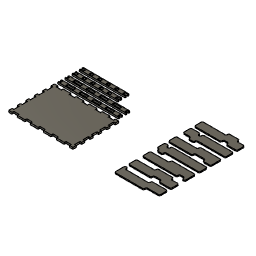
Púsl og Bakki (Autodesk Fusion 360 design; units mm, degrees)
Autodesk Fusion 360 part; units mm, degrees
(part 1 of 3)
sketch "Sketch1" plane through (0, 0, 0) normal (0, 0, 1) x (1, 0, 0)
  line L0 (0, 0) -> (121.4, 0)
  line L1 (121.4, 0) -> (121.4, 86.4)
  line L2 (121.4, 86.4) -> (0, 86.4)
  line L3 (0, 86.4) -> (0, 0)
  line L4 (6.4, 0) -> (16.4, 0)
  line L5 (16.4, 0) -> (16.4, 3.2)
  line L6 (16.4, 3.2) -> (6.4, 3.2)
  line L7 (6.4, 3.2) -> (6.4, 0)
  line L8 (31.05, 3.2) -> (31.05, 0)
  line L9 (41.05, 3.2) -> (31.05, 3.2)
  line L10 (31.05, 0) -> (41.05, 0)
  line L11 (41.05, 0) -> (41.05, 3.2)
  line L12 (55.7, 3.2) -> (55.7, 0)
  line L13 (65.7, 3.2) -> (55.7, 3.2)
  line L14 (55.7, 0) -> (65.7, 0)
  line L15 (65.7, 0) -> (65.7, 3.2)
  line L16 (80.35, 3.2) -> (80.35, 0)
  line L17 (90.35, 3.2) -> (80.35, 3.2)
  line L18 (80.35, 0) -> (90.35, 0)
  line L19 (90.35, 0) -> (90.35, 3.2)
  line L20 (105, 3.2) -> (105, 0)
  line L21 (115, 3.2) -> (105, 3.2)
  line L22 (105, 0) -> (115, 0)
  line L23 (115, 0) -> (115, 3.2)
  line L24 (65.7, 83.2) -> (65.7, 86.4)
  line L25 (90.35, 86.4) -> (80.35, 86.4)
  line L26 (41.05, 83.2) -> (41.05, 86.4)
  line L27 (80.35, 86.4) -> (80.35, 83.2)
  line L28 (105, 83.2) -> (115, 83.2)
  line L29 (115, 86.4) -> (105, 86.4)
  line L30 (16.4, 83.2) -> (16.4, 86.4)
  line L31 (115, 83.2) -> (115, 86.4)
  line L32 (55.7, 83.2) -> (65.7, 83.2)
  line L33 (55.7, 86.4) -> (55.7, 83.2)
  line L34 (6.4, 86.4) -> (6.4, 83.2)
  line L35 (41.05, 86.4) -> (31.05, 86.4)
  line L36 (105, 86.4) -> (105, 83.2)
  line L37 (65.7, 86.4) -> (55.7, 86.4)
  line L38 (6.4, 83.2) -> (16.4, 83.2)
  line L39 (16.4, 86.4) -> (6.4, 86.4)
  line L40 (80.35, 83.2) -> (90.35, 83.2)
  line L41 (31.05, 86.4) -> (31.05, 83.2)
  line L42 (90.35, 83.2) -> (90.35, 86.4)
  line L43 (31.05, 83.2) -> (41.05, 83.2)
  line L44 (0, 6.4) -> (3.2, 6.4)
  line L45 (3.2, 6.4) -> (3.2, 16.4)
  line L46 (3.2, 16.4) -> (0, 16.4)
  line L47 (0, 16.4) -> (0, 6.4)
  line L48 (0, 22.3) -> (3.2, 22.3)
  line L49 (0, 32.3) -> (0, 22.3)
  line L50 (3.2, 22.3) -> (3.2, 32.3)
  line L51 (3.2, 32.3) -> (0, 32.3)
  line L52 (0, 38.2) -> (3.2, 38.2)
  line L53 (0, 48.2) -> (0, 38.2)
  line L54 (3.2, 38.2) -> (3.2, 48.2)
  line L55 (3.2, 48.2) -> (0, 48.2)
  line L56 (0, 54.1) -> (3.2, 54.1)
  line L57 (0, 64.1) -> (0, 54.1)
  line L58 (3.2, 54.1) -> (3.2, 64.1)
  line L59 (3.2, 64.1) -> (0, 64.1)
  line L60 (0, 70) -> (3.2, 70)
  line L61 (0, 80) -> (0, 70)
  line L62 (3.2, 70) -> (3.2, 80)
  line L63 (3.2, 80) -> (0, 80)
  line L64 (121.4, 70) -> (121.4, 80)
  line L65 (121.4, 16.4) -> (118.2, 16.4)
  line L66 (118.2, 16.4) -> (118.2, 6.4)
  line L67 (118.2, 38.2) -> (121.4, 38.2)
  line L68 (118.2, 54.1) -> (121.4, 54.1)
  line L69 (121.4, 22.3) -> (121.4, 32.3)
  line L70 (121.4, 6.4) -> (121.4, 16.4)
  line L71 (121.4, 48.2) -> (118.2, 48.2)
  line L72 (121.4, 54.1) -> (121.4, 64.1)
  line L73 (121.4, 64.1) -> (118.2, 64.1)
  line L74 (118.2, 64.1) -> (118.2, 54.1)
  line L75 (121.4, 38.2) -> (121.4, 48.2)
  line L76 (118.2, 80) -> (118.2, 70)
  line L77 (121.4, 80) -> (118.2, 80)
  line L78 (118.2, 22.3) -> (121.4, 22.3)
  line L79 (121.4, 32.3) -> (118.2, 32.3)
  line L80 (118.2, 70) -> (121.4, 70)
  line L81 (118.2, 6.4) -> (121.4, 6.4)
  line L82 (118.2, 48.2) -> (118.2, 38.2)
  line L83 (118.2, 32.3) -> (118.2, 22.3)
  dimension "d1" = 121.4
  dimension "d2" = 86.4
  dimension "d6" = 10
  dimension "d7" = 3.2
  dimension "d8" = 6.4
  dimension "d12" = 98.6
  dimension "d13" = 0
  dimension "d16" = 0
  dimension "d17" = 83.2
  dimension "d18" = 3.2
  dimension "d19" = 10
  dimension "d20" = 6.4
  dimension "d23" = 0
  dimension "d24" = 63.6
  dimension "d27" = 118.2
  dimension "d28" = 0
  constraint horizontal L0
  constraint vertical L1
  constraint horizontal L2
  constraint coincident L0.start L3.end
  constraint horizontal L4
  constraint vertical L5
  constraint horizontal L6
  constraint vertical L7
  constraint coincident L0 L4.start
  constraint horizontal L44
  constraint vertical L45
  constraint horizontal L46
  constraint vertical L47
  constraint coincident L3 L44.start
  measures "d1" distance of L0.start L0.end
  measures "d2" distance of L0.start L2.end
  measures "d6" distance of L4.start L4.end
  measures "d7" distance of L4.start L6.end
  measures "d8" distance of L3 L7
  measures "d18" distance of L44.start L44.end
  measures "d19" distance of L44.start L46.end
  measures "d20" distance of L0 L44
extrude "Extrude1" add sketch "Sketch1" along normal blind 3.2 contours L0 L1 L2 L3 L5 L6 L7 L8 L9 L11 L12 L13 L15 L16 L17 L19 L20 L21 L23 L24 L26 L27 L28 L30 L31 L32 L33 L34 L36 L38 L40 L41 L42 L43 L44 L45 L46 L48 L50 L51 L52 L54 L55 L56 L58 L59 L60 L62 L63 L65 L66 L67 L68 L71 L73 L74 L76 L77 L78 L79 L80 L81 L82 L83 makes body 1
sketch "Sketch13" plane through (0, 0, 3.2) normal (0, 0, 1) x (-1, 0, 0)
  line L0 (-121.4, -32.3) -> (-121.4, -38.2)
  line L1 (-121.4, -38.2) -> (-118.2, -38.2)
  line L2 (-118.2, -38.2) -> (-118.2, -48.2)
  line L3 (-118.2, -48.2) -> (-121.4, -48.2)
  line L4 (-121.4, -48.2) -> (-121.4, -54.1)
  line L5 (-121.4, -54.1) -> (-118.2, -54.1)
  line L6 (-118.2, -54.1) -> (-118.2, -64.1)
  line L7 (-118.2, -64.1) -> (-121.4, -64.1)
  line L8 (-121.4, -64.1) -> (-121.4, -70)
  line L9 (-121.4, -70) -> (-118.2, -70)
  line L10 (-118.2, -70) -> (-118.2, -80)
  line L11 (-118.2, -80) -> (-121.4, -80)
  line L12 (-121.4, -80) -> (-121.4, -86.4)
  line L13 (-121.4, -86.4) -> (-115, -86.4)
  line L14 (-115, -86.4) -> (-115, -83.2)
  line L15 (-115, -83.2) -> (-105, -83.2)
  line L16 (-105, -83.2) -> (-105, -86.4)
  line L17 (-105, -86.4) -> (-90.35, -86.4)
  line L18 (-90.35, -86.4) -> (-90.35, -83.2)
  line L19 (-90.35, -83.2) -> (-80.35, -83.2)
  line L20 (-80.35, -83.2) -> (-80.35, -86.4)
  line L21 (-80.35, -86.4) -> (-65.7, -86.4)
  line L22 (-65.7, -86.4) -> (-65.7, -83.2)
  line L23 (-65.7, -83.2) -> (-55.7, -83.2)
  line L24 (-55.7, -83.2) -> (-55.7, -86.4)
  line L25 (-55.7, -86.4) -> (-41.05, -86.4)
  line L26 (-41.05, -86.4) -> (-41.05, -83.2)
  line L27 (-41.05, -83.2) -> (-31.05, -83.2)
  line L28 (-31.05, -83.2) -> (-31.05, -86.4)
  line L29 (-31.05, -86.4) -> (-16.4, -86.4)
  line L30 (-16.4, -86.4) -> (-16.4, -83.2)
  line L31 (-16.4, -83.2) -> (-6.4, -83.2)
  line L32 (-6.4, -83.2) -> (-6.4, -86.4)
  line L33 (-6.4, -86.4) -> (0, -86.4)
  line L34 (0, -86.4) -> (0, -80)
  line L35 (0, -80) -> (-3.2, -80)
  line L36 (-3.2, -80) -> (-3.2, -70)
  line L37 (-3.2, -70) -> (0, -70)
  line L38 (0, -70) -> (0, -64.1)
  line L39 (0, -64.1) -> (-3.2, -64.1)
  line L40 (-3.2, -64.1) -> (-3.2, -54.1)
  line L41 (-3.2, -54.1) -> (0, -54.1)
  line L42 (0, -54.1) -> (0, -48.2)
  line L43 (0, -48.2) -> (-3.2, -48.2)
  line L44 (-3.2, -48.2) -> (-3.2, -38.2)
  line L45 (-3.2, -38.2) -> (0, -38.2)
  line L46 (0, -38.2) -> (0, -32.3)
  line L47 (0, -32.3) -> (-3.2, -32.3)
  line L48 (-3.2, -32.3) -> (-3.2, -22.3)
  line L49 (-3.2, -22.3) -> (0, -22.3)
  line L50 (0, -22.3) -> (0, -16.4)
  line L51 (0, -16.4) -> (-3.2, -16.4)
  line L52 (-3.2, -16.4) -> (-3.2, -6.4)
  line L53 (-3.2, -6.4) -> (0, -6.4)
  line L54 (0, -6.4) -> (0, 0)
  line L55 (0, 0) -> (-6.4, 0)
  line L56 (-6.4, 0) -> (-6.4, -3.2)
  line L57 (-6.4, -3.2) -> (-16.4, -3.2)
  line L58 (-16.4, -3.2) -> (-16.4, 0)
  line L59 (-16.4, 0) -> (-31.05, 0)
  line L60 (-31.05, 0) -> (-31.05, -3.2)
  line L61 (-31.05, -3.2) -> (-41.05, -3.2)
  line L62 (-41.05, -3.2) -> (-41.05, 0)
  line L63 (-41.05, 0) -> (-55.7, 0)
  line L64 (-55.7, 0) -> (-55.7, -3.2)
  line L65 (-55.7, -3.2) -> (-65.7, -3.2)
  line L66 (-65.7, -3.2) -> (-65.7, 0)
  line L67 (-65.7, 0) -> (-80.35, 0)
  line L68 (-80.35, 0) -> (-80.35, -3.2)
  line L69 (-80.35, -3.2) -> (-90.35, -3.2)
  line L70 (-90.35, -3.2) -> (-90.35, 0)
  line L71 (-90.35, 0) -> (-105, 0)
  line L72 (-105, 0) -> (-105, -3.2)
  line L73 (-105, -3.2) -> (-115, -3.2)
  line L74 (-115, -3.2) -> (-115, 0)
  line L75 (-115, 0) -> (-121.4, 0)
  line L76 (-121.4, 0) -> (-121.4, -6.4)
  line L77 (-121.4, -6.4) -> (-118.2, -6.4)
  line L78 (-118.2, -6.4) -> (-118.2, -16.4)
  line L79 (-118.2, -16.4) -> (-121.4, -16.4)
  line L80 (-121.4, -16.4) -> (-121.4, -22.3)
  line L81 (-121.4, -22.3) -> (-118.2, -22.3)
  line L82 (-118.2, -22.3) -> (-118.2, -32.3)
  line L83 (-118.2, -32.3) -> (-121.4, -32.3)
  line L84 (0, 0) -> (-3.2, 0)
  line L85 (-3.2, 0) -> (-3.2, -86.4)
  line L86 (-3.2, -86.4) -> (0, -86.4)
  line L87 (0, -86.4) -> (0, 0)
  dimension "d74" = 3.2
  dimension "d75" = 86.4
  constraint horizontal L84
  constraint vertical L85
  constraint horizontal L86
  constraint vertical L87
  constraint coincident L54.end L55.start
  measures "d74" distance of L54.end L84.end
  measures "d75" distance of L54.end L33.end
extrude "Extrude14" add sketch "Sketch13" against normal blind 3.2 separate body contours L51 L52 L53 L85 L87 | L47 L48 L49 L85 L87 | L43 L44 L45 L85 L87 | L35 L36 L37 L85 L87 | L39 L40 L41 L85 L87 makes body 2 at (1.0667, 41.5333, 3.2) makes body 3 at (2.1333, 57.4333, 3.2) makes body 4 at (2.1333, 25.6333, 3.2) makes body 5 at (3.2, 73.3333, 2.1333) makes body 6 at (2.1333, 9.7333, 3.2)
sketch "Sketch14" plane through (0, 0, 3.2) normal (0, 0, 1) x (-1, 0, 0)
  line L0 (-121.4, -32.3) -> (-121.4, -38.2)
  line L1 (-121.4, -38.2) -> (-118.2, -38.2)
  line L2 (-118.2, -38.2) -> (-118.2, -48.2)
  line L3 (-118.2, -48.2) -> (-121.4, -48.2)
  line L4 (-121.4, -48.2) -> (-121.4, -54.1)
  line L5 (-121.4, -54.1) -> (-118.2, -54.1)
  line L6 (-118.2, -54.1) -> (-118.2, -64.1)
  line L7 (-118.2, -64.1) -> (-121.4, -64.1)
  line L8 (-121.4, -64.1) -> (-121.4, -70)
  line L9 (-121.4, -70) -> (-118.2, -70)
  line L10 (-118.2, -70) -> (-118.2, -80)
  line L11 (-118.2, -80) -> (-121.4, -80)
  line L12 (-121.4, -80) -> (-121.4, -86.4)
  line L13 (-121.4, -86.4) -> (-115, -86.4)
  line L14 (-115, -86.4) -> (-115, -83.2)
  line L15 (-115, -83.2) -> (-105, -83.2)
  line L16 (-105, -83.2) -> (-105, -86.4)
  line L17 (-105, -86.4) -> (-90.35, -86.4)
  line L18 (-90.35, -86.4) -> (-90.35, -83.2)
  line L19 (-90.35, -83.2) -> (-80.35, -83.2)
  line L20 (-80.35, -83.2) -> (-80.35, -86.4)
  line L21 (-80.35, -86.4) -> (-65.7, -86.4)
  line L22 (-65.7, -86.4) -> (-65.7, -83.2)
  line L23 (-65.7, -83.2) -> (-55.7, -83.2)
  line L24 (-55.7, -83.2) -> (-55.7, -86.4)
  line L25 (-55.7, -86.4) -> (-41.05, -86.4)
  line L26 (-41.05, -86.4) -> (-41.05, -83.2)
  line L27 (-41.05, -83.2) -> (-31.05, -83.2)
  line L28 (-31.05, -83.2) -> (-31.05, -86.4)
  line L29 (-31.05, -86.4) -> (-16.4, -86.4)
  line L30 (-16.4, -86.4) -> (-16.4, -83.2)
  line L31 (-16.4, -83.2) -> (-6.4, -83.2)
  line L32 (-6.4, -83.2) -> (-6.4, -86.4)
  line L33 (-6.4, -86.4) -> (0, -86.4)
  line L34 (0, -86.4) -> (0, -80)
  line L35 (0, -80) -> (-3.2, -80)
  line L36 (-3.2, -80) -> (-3.2, -70)
  line L37 (-3.2, -70) -> (0, -70)
  line L38 (0, -70) -> (0, -64.1)
  line L39 (0, -64.1) -> (-3.2, -64.1)
  line L40 (-3.2, -64.1) -> (-3.2, -54.1)
  line L41 (-3.2, -54.1) -> (0, -54.1)
  line L42 (0, -54.1) -> (0, -48.2)
  line L43 (0, -48.2) -> (-3.2, -48.2)
  line L44 (-3.2, -48.2) -> (-3.2, -38.2)
  line L45 (-3.2, -38.2) -> (0, -38.2)
  line L46 (0, -38.2) -> (0, -32.3)
  line L47 (0, -32.3) -> (-3.2, -32.3)
  line L48 (-3.2, -32.3) -> (-3.2, -22.3)
  line L49 (-3.2, -22.3) -> (0, -22.3)
  line L50 (0, -22.3) -> (0, -16.4)
  line L51 (0, -16.4) -> (-3.2, -16.4)
  line L52 (-3.2, -16.4) -> (-3.2, -6.4)
  line L53 (-3.2, -6.4) -> (0, -6.4)
  line L54 (0, -6.4) -> (0, 0)
  line L55 (0, 0) -> (-6.4, 0)
  line L56 (-6.4, 0) -> (-6.4, -3.2)
  line L57 (-6.4, -3.2) -> (-16.4, -3.2)
  line L58 (-16.4, -3.2) -> (-16.4, 0)
  line L59 (-16.4, 0) -> (-31.05, 0)
  line L60 (-31.05, 0) -> (-31.05, -3.2)
  line L61 (-31.05, -3.2) -> (-41.05, -3.2)
  line L62 (-41.05, -3.2) -> (-41.05, 0)
  line L63 (-41.05, 0) -> (-55.7, 0)
  line L64 (-55.7, 0) -> (-55.7, -3.2)
  line L65 (-55.7, -3.2) -> (-65.7, -3.2)
  line L66 (-65.7, -3.2) -> (-65.7, 0)
  line L67 (-65.7, 0) -> (-80.35, 0)
  line L68 (-80.35, 0) -> (-80.35, -3.2)
  line L69 (-80.35, -3.2) -> (-90.35, -3.2)
  line L70 (-90.35, -3.2) -> (-90.35, 0)
  line L71 (-90.35, 0) -> (-105, 0)
  line L72 (-105, 0) -> (-105, -3.2)
  line L73 (-105, -3.2) -> (-115, -3.2)
  line L74 (-115, -3.2) -> (-115, 0)
  line L75 (-115, 0) -> (-121.4, 0)
  line L76 (-121.4, 0) -> (-121.4, -6.4)
  line L77 (-121.4, -6.4) -> (-118.2, -6.4)
  line L78 (-118.2, -6.4) -> (-118.2, -16.4)
  line L79 (-118.2, -16.4) -> (-121.4, -16.4)
  line L80 (-121.4, -16.4) -> (-121.4, -22.3)
  line L81 (-121.4, -22.3) -> (-118.2, -22.3)
  line L82 (-118.2, -22.3) -> (-118.2, -32.3)
  line L83 (-118.2, -32.3) -> (-121.4, -32.3)
  line L84 (0, 0) -> (-3.2, 0)
  line L85 (-3.2, 0) -> (-3.2, -86.4)
  line L86 (-3.2, -86.4) -> (0, -86.4)
  line L87 (0, -86.4) -> (0, 0)
  dimension "d78" = 3.2
  dimension "d79" = 86.4
  constraint horizontal L84
  constraint vertical L85
  constraint horizontal L86
  constraint vertical L87
  constraint coincident L54.end L55.start
  measures "d78" distance of L54.end L84.end
  measures "d79" distance of L54.end L33.end
extrude "Extrude15" add sketch "Sketch14" along normal blind 2 contours L53 L54 L55 L84 L85 L87 | L51 L52 L53 L85 L87 | L49 L50 L51 L85 L87 | L47 L48 L49 L85 L87 | L45 L46 L47 L85 L87 | L33 L34 L35 L85 L86 L87 | L43 L44 L45 L85 L87 | L35 L36 L37 L85 L87 | L41 L42 L43 L85 L87 | L37 L38 L39 L85 L87 | L39 L40 L41 L85 L87 bodies 2 3 4 5 6
sketch "Sketch15" plane through (0, 0, 0) normal (0, 0, -1) x (1, 0, 0)
  line L0 (121.4, -38.2) -> (121.4, -32.3)
  line L1 (121.4, -32.3) -> (118.2, -32.3)
  line L2 (118.2, -32.3) -> (118.2, -22.3)
  line L3 (118.2, -22.3) -> (121.4, -22.3)
  line L4 (121.4, -22.3) -> (121.4, -16.4)
  line L5 (121.4, -16.4) -> (118.2, -16.4)
  line L6 (118.2, -16.4) -> (118.2, -6.4)
  line L7 (118.2, -6.4) -> (121.4, -6.4)
  line L8 (121.4, -6.4) -> (121.4, 0)
  line L9 (121.4, 0) -> (115, 0)
  line L10 (115, 0) -> (115, -3.2)
  line L11 (115, -3.2) -> (105, -3.2)
  line L12 (105, -3.2) -> (105, 0)
  line L13 (105, 0) -> (90.35, 0)
  line L14 (90.35, 0) -> (90.35, -3.2)
  line L15 (90.35, -3.2) -> (80.35, -3.2)
  line L16 (80.35, -3.2) -> (80.35, 0)
  line L17 (80.35, 0) -> (65.7, 0)
  line L18 (65.7, 0) -> (65.7, -3.2)
  line L19 (65.7, -3.2) -> (55.7, -3.2)
  line L20 (55.7, -3.2) -> (55.7, 0)
  line L21 (55.7, 0) -> (41.05, 0)
  line L22 (41.05, 0) -> (41.05, -3.2)
  line L23 (41.05, -3.2) -> (31.05, -3.2)
  line L24 (31.05, -3.2) -> (31.05, 0)
  line L25 (31.05, 0) -> (16.4, 0)
  line L26 (16.4, 0) -> (16.4, -3.2)
  line L27 (16.4, -3.2) -> (6.4, -3.2)
  line L28 (6.4, -3.2) -> (6.4, 0)
  line L29 (6.4, 0) -> (0, 0)
  line L30 (0, 0) -> (0, -6.4)
  line L31 (0, -6.4) -> (3.2, -6.4)
  line L32 (3.2, -6.4) -> (3.2, -16.4)
  line L33 (3.2, -16.4) -> (0, -16.4)
  line L34 (0, -16.4) -> (0, -22.3)
  line L35 (0, -22.3) -> (3.2, -22.3)
  line L36 (3.2, -22.3) -> (3.2, -32.3)
  line L37 (3.2, -32.3) -> (0, -32.3)
  line L38 (0, -32.3) -> (0, -38.2)
  line L39 (0, -38.2) -> (3.2, -38.2)
  line L40 (3.2, -38.2) -> (3.2, -48.2)
  line L41 (3.2, -48.2) -> (0, -48.2)
  line L42 (0, -48.2) -> (0, -54.1)
  line L43 (0, -54.1) -> (3.2, -54.1)
  line L44 (3.2, -54.1) -> (3.2, -64.1)
  line L45 (3.2, -64.1) -> (0, -64.1)
  line L46 (0, -64.1) -> (0, -70)
  line L47 (0, -70) -> (3.2, -70)
  line L48 (3.2, -70) -> (3.2, -80)
  line L49 (3.2, -80) -> (0, -80)
  line L50 (0, -80) -> (0, -86.4)
  line L51 (0, -86.4) -> (6.4, -86.4)
  line L52 (6.4, -86.4) -> (6.4, -83.2)
  line L53 (6.4, -83.2) -> (16.4, -83.2)
  line L54 (16.4, -83.2) -> (16.4, -86.4)
  line L55 (16.4, -86.4) -> (31.05, -86.4)
  line L56 (31.05, -86.4) -> (31.05, -83.2)
  line L57 (31.05, -83.2) -> (41.05, -83.2)
  line L58 (41.05, -83.2) -> (41.05, -86.4)
  line L59 (41.05, -86.4) -> (55.7, -86.4)
  line L60 (55.7, -86.4) -> (55.7, -83.2)
  line L61 (55.7, -83.2) -> (65.7, -83.2)
  line L62 (65.7, -83.2) -> (65.7, -86.4)
  line L63 (65.7, -86.4) -> (80.35, -86.4)
  line L64 (80.35, -86.4) -> (80.35, -83.2)
  line L65 (80.35, -83.2) -> (90.35, -83.2)
  line L66 (90.35, -83.2) -> (90.35, -86.4)
  line L67 (90.35, -86.4) -> (105, -86.4)
  line L68 (105, -86.4) -> (105, -83.2)
  line L69 (105, -83.2) -> (115, -83.2)
  line L70 (115, -83.2) -> (115, -86.4)
  line L71 (115, -86.4) -> (121.4, -86.4)
  line L72 (121.4, -86.4) -> (121.4, -80)
  line L73 (121.4, -80) -> (118.2, -80)
  line L74 (118.2, -80) -> (118.2, -70)
  line L75 (118.2, -70) -> (121.4, -70)
  line L76 (121.4, -70) -> (121.4, -64.1)
  line L77 (121.4, -64.1) -> (118.2, -64.1)
  line L78 (118.2, -64.1) -> (118.2, -54.1)
  line L79 (118.2, -54.1) -> (121.4, -54.1)
  line L80 (121.4, -54.1) -> (121.4, -48.2)
  line L81 (121.4, -48.2) -> (118.2, -48.2)
  line L82 (118.2, -48.2) -> (118.2, -38.2)
  line L83 (118.2, -38.2) -> (121.4, -38.2)
  line L84 (0, 0) -> (3.2, 0)
  line L85 (3.2, 0) -> (3.2, -86.4)
  line L86 (3.2, -86.4) -> (0, -86.4)
  line L87 (0, -86.4) -> (0, 0)
  dimension "d82" = 3.2
  dimension "d83" = 86.4
  constraint horizontal L84
  constraint vertical L85
  constraint horizontal L86
  constraint vertical L87
  constraint coincident L29.end L30.start
  measures "d82" distance of L29.end L84.end
  measures "d83" distance of L29.end L50.end
extrude "Extrude16" add sketch "Sketch15" along normal blind 2 contours L29 L30 L31 L84 L85 L87 | L31 L32 L33 L85 L87 | L33 L34 L35 L85 L87 | L35 L36 L37 L85 L87 | L49 L50 L51 L85 L86 L87 | L37 L38 L39 L85 L87 | L47 L48 L49 L85 L87 | L39 L40 L41 L85 L87 | L45 L46 L47 L85 L87 | L41 L42 L43 L85 L87 | L43 L44 L45 L85 L87 bodies 2
sketch "Sketch16" plane through (0, 0, 3.2) normal (0, 0, 1) x (-1, 0, 0)
  line L0 (-121.4, -32.3) -> (-121.4, -38.2)
  line L1 (-121.4, -38.2) -> (-118.2, -38.2)
  line L2 (-118.2, -38.2) -> (-118.2, -48.2)
  line L3 (-118.2, -48.2) -> (-121.4, -48.2)
  line L4 (-121.4, -48.2) -> (-121.4, -54.1)
  line L5 (-121.4, -54.1) -> (-118.2, -54.1)
  line L6 (-118.2, -54.1) -> (-118.2, -64.1)
  line L7 (-118.2, -64.1) -> (-121.4, -64.1)
  line L8 (-121.4, -64.1) -> (-121.4, -70)
  line L9 (-121.4, -70) -> (-118.2, -70)
  line L10 (-118.2, -70) -> (-118.2, -80)
  line L11 (-118.2, -80) -> (-121.4, -80)
  line L12 (-121.4, -80) -> (-121.4, -86.4)
  line L13 (-121.4, -86.4) -> (-115, -86.4)
  line L14 (-115, -86.4) -> (-115, -83.2)
  line L15 (-115, -83.2) -> (-105, -83.2)
  line L16 (-105, -83.2) -> (-105, -86.4)
  line L17 (-105, -86.4) -> (-90.35, -86.4)
  line L18 (-90.35, -86.4) -> (-90.35, -83.2)
  line L19 (-90.35, -83.2) -> (-80.35, -83.2)
  line L20 (-80.35, -83.2) -> (-80.35, -86.4)
  line L21 (-80.35, -86.4) -> (-65.7, -86.4)
  line L22 (-65.7, -86.4) -> (-65.7, -83.2)
  line L23 (-65.7, -83.2) -> (-55.7, -83.2)
  line L24 (-55.7, -83.2) -> (-55.7, -86.4)
  line L25 (-55.7, -86.4) -> (-41.05, -86.4)
  line L26 (-41.05, -86.4) -> (-41.05, -83.2)
  line L27 (-41.05, -83.2) -> (-31.05, -83.2)
  line L28 (-31.05, -83.2) -> (-31.05, -86.4)
  line L29 (-31.05, -86.4) -> (-16.4, -86.4)
  line L30 (-16.4, -86.4) -> (-16.4, -83.2)
  line L31 (-16.4, -83.2) -> (-6.4, -83.2)
  line L32 (-6.4, -83.2) -> (-6.4, -86.4)
  line L33 (-6.4, -86.4) -> (0, -86.4)
  line L34 (0, -86.4) -> (0, -80)
  line L35 (0, -80) -> (-3.2, -80)
  line L36 (-3.2, -80) -> (-3.2, -70)
  line L37 (-3.2, -70) -> (0, -70)
  line L38 (0, -70) -> (0, -64.1)
  line L39 (0, -64.1) -> (-3.2, -64.1)
  line L40 (-3.2, -64.1) -> (-3.2, -54.1)
  line L41 (-3.2, -54.1) -> (0, -54.1)
  line L42 (0, -54.1) -> (0, -48.2)
  line L43 (0, -48.2) -> (-3.2, -48.2)
  line L44 (-3.2, -48.2) -> (-3.2, -38.2)
  line L45 (-3.2, -38.2) -> (0, -38.2)
  line L46 (0, -38.2) -> (0, -32.3)
  line L47 (0, -32.3) -> (-3.2, -32.3)
  line L48 (-3.2, -32.3) -> (-3.2, -22.3)
  line L49 (-3.2, -22.3) -> (0, -22.3)
  line L50 (0, -22.3) -> (0, -16.4)
  line L51 (0, -16.4) -> (-3.2, -16.4)
  line L52 (-3.2, -16.4) -> (-3.2, -6.4)
  line L53 (-3.2, -6.4) -> (0, -6.4)
  line L54 (0, -6.4) -> (0, 0)
  line L55 (0, 0) -> (-6.4, 0)
  line L56 (-6.4, 0) -> (-6.4, -3.2)
  line L57 (-6.4, -3.2) -> (-16.4, -3.2)
  line L58 (-16.4, -3.2) -> (-16.4, 0)
  line L59 (-16.4, 0) -> (-31.05, 0)
  line L60 (-31.05, 0) -> (-31.05, -3.2)
  line L61 (-31.05, -3.2) -> (-41.05, -3.2)
  line L62 (-41.05, -3.2) -> (-41.05, 0)
  line L63 (-41.05, 0) -> (-55.7, 0)
  line L64 (-55.7, 0) -> (-55.7, -3.2)
  line L65 (-55.7, -3.2) -> (-65.7, -3.2)
  line L66 (-65.7, -3.2) -> (-65.7, 0)
  line L67 (-65.7, 0) -> (-80.35, 0)
  line L68 (-80.35, 0) -> (-80.35, -3.2)
  line L69 (-80.35, -3.2) -> (-90.35, -3.2)
  line L70 (-90.35, -3.2) -> (-90.35, 0)
  line L71 (-90.35, 0) -> (-105, 0)
  line L72 (-105, 0) -> (-105, -3.2)
  line L73 (-105, -3.2) -> (-115, -3.2)
  line L74 (-115, -3.2) -> (-115, 0)
  line L75 (-115, 0) -> (-121.4, 0)
  line L76 (-121.4, 0) -> (-121.4, -6.4)
  line L77 (-121.4, -6.4) -> (-118.2, -6.4)
  line L78 (-118.2, -6.4) -> (-118.2, -16.4)
  line L79 (-118.2, -16.4) -> (-121.4, -16.4)
  line L80 (-121.4, -16.4) -> (-121.4, -22.3)
  line L81 (-121.4, -22.3) -> (-118.2, -22.3)
  line L82 (-118.2, -22.3) -> (-118.2, -32.3)
  line L83 (-118.2, -32.3) -> (-121.4, -32.3)
  line L84 (-3.2, 0) -> (-118.2, 0)
  line L85 (-118.2, 0) -> (-118.2, -3.2)
  line L86 (-118.2, -3.2) -> (-3.2, -3.2)
  line L87 (-3.2, -3.2) -> (-3.2, 0)
  dimension "d86" = 115
  dimension "d87" = 3.2
  constraint horizontal L84
  constraint vertical L85
  constraint horizontal L86
  constraint vertical L87
  constraint midpoint L55 L84.start
  measures "d86" distance of L84.start L84.end
  measures "d87" distance of L84.start L86.end
extrude "Extrude17" add sketch "Sketch16" against normal blind 3.2 separate body contours L72 L73 L74 L84 L86 | L68 L69 L70 L84 L86 | L64 L65 L66 L84 L86 | L60 L61 L62 L84 L86 | L56 L57 L58 L84 L86 makes body 7 at (62.3667, 3.2, 1.0667) makes body 8 at (87.0167, 0, 1.0667) makes body 9 at (37.7167, 3.2, 1.0667) makes body 10 at (111.6667, 0, 1.0667) makes body 11 at (13.0667, 0, 1.0667)
sketch "Sketch17" plane through (0, 0, 3.2) normal (0, 0, 1) x (-1, 0, 0)
  line L0 (-121.4, -32.3) -> (-121.4, -38.2)
  line L1 (-121.4, -38.2) -> (-118.2, -38.2)
  line L2 (-118.2, -38.2) -> (-118.2, -48.2)
  line L3 (-118.2, -48.2) -> (-121.4, -48.2)
  line L4 (-121.4, -48.2) -> (-121.4, -54.1)
  line L5 (-121.4, -54.1) -> (-118.2, -54.1)
  line L6 (-118.2, -54.1) -> (-118.2, -64.1)
  line L7 (-118.2, -64.1) -> (-121.4, -64.1)
  line L8 (-121.4, -64.1) -> (-121.4, -70)
  line L9 (-121.4, -70) -> (-118.2, -70)
  line L10 (-118.2, -70) -> (-118.2, -80)
  line L11 (-118.2, -80) -> (-121.4, -80)
  line L12 (-121.4, -80) -> (-121.4, -86.4)
  line L13 (-121.4, -86.4) -> (-115, -86.4)
  line L14 (-115, -86.4) -> (-115, -83.2)
  line L15 (-115, -83.2) -> (-105, -83.2)
  line L16 (-105, -83.2) -> (-105, -86.4)
  line L17 (-105, -86.4) -> (-90.35, -86.4)
  line L18 (-90.35, -86.4) -> (-90.35, -83.2)
  line L19 (-90.35, -83.2) -> (-80.35, -83.2)
  line L20 (-80.35, -83.2) -> (-80.35, -86.4)
  line L21 (-80.35, -86.4) -> (-65.7, -86.4)
  line L22 (-65.7, -86.4) -> (-65.7, -83.2)
  line L23 (-65.7, -83.2) -> (-55.7, -83.2)
  line L24 (-55.7, -83.2) -> (-55.7, -86.4)
  line L25 (-55.7, -86.4) -> (-41.05, -86.4)
  line L26 (-41.05, -86.4) -> (-41.05, -83.2)
  line L27 (-41.05, -83.2) -> (-31.05, -83.2)
  line L28 (-31.05, -83.2) -> (-31.05, -86.4)
  line L29 (-31.05, -86.4) -> (-16.4, -86.4)
  line L30 (-16.4, -86.4) -> (-16.4, -83.2)
  line L31 (-16.4, -83.2) -> (-6.4, -83.2)
  line L32 (-6.4, -83.2) -> (-6.4, -86.4)
  line L33 (-6.4, -86.4) -> (0, -86.4)
  line L34 (0, -86.4) -> (0, -80)
  line L35 (0, -80) -> (-3.2, -80)
  line L36 (-3.2, -80) -> (-3.2, -70)
  line L37 (-3.2, -70) -> (0, -70)
  line L38 (0, -70) -> (0, -64.1)
  line L39 (0, -64.1) -> (-3.2, -64.1)
  line L40 (-3.2, -64.1) -> (-3.2, -54.1)
  line L41 (-3.2, -54.1) -> (0, -54.1)
  line L42 (0, -54.1) -> (0, -48.2)
  line L43 (0, -48.2) -> (-3.2, -48.2)
  line L44 (-3.2, -48.2) -> (-3.2, -38.2)
  line L45 (-3.2, -38.2) -> (0, -38.2)
  line L46 (0, -38.2) -> (0, -32.3)
  line L47 (0, -32.3) -> (-3.2, -32.3)
  line L48 (-3.2, -32.3) -> (-3.2, -22.3)
  line L49 (-3.2, -22.3) -> (0, -22.3)
  line L50 (0, -22.3) -> (0, -16.4)
  line L51 (0, -16.4) -> (-3.2, -16.4)
  line L52 (-3.2, -16.4) -> (-3.2, -6.4)
  line L53 (-3.2, -6.4) -> (0, -6.4)
  line L54 (0, -6.4) -> (0, 0)
  line L55 (0, 0) -> (-6.4, 0)
  line L56 (-6.4, 0) -> (-6.4, -3.2)
  line L57 (-6.4, -3.2) -> (-16.4, -3.2)
  line L58 (-16.4, -3.2) -> (-16.4, 0)
  line L59 (-16.4, 0) -> (-31.05, 0)
  line L60 (-31.05, 0) -> (-31.05, -3.2)
  line L61 (-31.05, -3.2) -> (-41.05, -3.2)
  line L62 (-41.05, -3.2) -> (-41.05, 0)
  line L63 (-41.05, 0) -> (-55.7, 0)
  line L64 (-55.7, 0) -> (-55.7, -3.2)
  line L65 (-55.7, -3.2) -> (-65.7, -3.2)
  line L66 (-65.7, -3.2) -> (-65.7, 0)
  line L67 (-65.7, 0) -> (-80.35, 0)
  line L68 (-80.35, 0) -> (-80.35, -3.2)
  line L69 (-80.35, -3.2) -> (-90.35, -3.2)
  line L70 (-90.35, -3.2) -> (-90.35, 0)
  line L71 (-90.35, 0) -> (-105, 0)
  line L72 (-105, 0) -> (-105, -3.2)
  line L73 (-105, -3.2) -> (-115, -3.2)
  line L74 (-115, -3.2) -> (-115, 0)
  line L75 (-115, 0) -> (-121.4, 0)
  line L76 (-121.4, 0) -> (-121.4, -6.4)
  line L77 (-121.4, -6.4) -> (-118.2, -6.4)
  line L78 (-118.2, -6.4) -> (-118.2, -16.4)
  line L79 (-118.2, -16.4) -> (-121.4, -16.4)
  line L80 (-121.4, -16.4) -> (-121.4, -22.3)
  line L81 (-121.4, -22.3) -> (-118.2, -22.3)
  line L82 (-118.2, -22.3) -> (-118.2, -32.3)
  line L83 (-118.2, -32.3) -> (-121.4, -32.3)
  line L84 (-118.2, 0) -> (-3.2, 0)
  line L85 (-3.2, 0) -> (-3.2, -3.2)
  line L86 (-3.2, -3.2) -> (-118.2, -3.2)
  line L87 (-118.2, -3.2) -> (-118.2, 0)
  dimension "d90" = 115
  dimension "d91" = 3.2
  constraint horizontal L84
  constraint vertical L85
  constraint horizontal L86
  constraint vertical L87
  constraint midpoint L75 L84.start
  measures "d90" distance of L84.start L84.end
  measures "d91" distance of L84.start L86.end
extrude "Extrude18" add sketch "Sketch17" along normal blind 2 contours L74 L75 L84 L86 L87 | L72 L73 L74 L84 L86 | L70 L71 L72 L84 L86 | L68 L69 L70 L84 L86 | L66 L67 L68 L84 L86 | L64 L65 L66 L84 L86 | L62 L63 L64 L84 L86 | L60 L61 L62 L84 L86 | L58 L59 L60 L84 L86 | L56 L57 L58 L84 L86 | L55 L56 L84 L85 L86 bodies 7 8 9 10 11
sketch "Sketch18" plane through (0, 0, 0) normal (0, 0, -1) x (1, 0, 0)
  line L0 (121.4, -38.2) -> (121.4, -32.3)
  line L1 (121.4, -32.3) -> (118.2, -32.3)
  line L2 (118.2, -32.3) -> (118.2, -22.3)
  line L3 (118.2, -22.3) -> (121.4, -22.3)
  line L4 (121.4, -22.3) -> (121.4, -16.4)
  line L5 (121.4, -16.4) -> (118.2, -16.4)
  line L6 (118.2, -16.4) -> (118.2, -6.4)
  line L7 (118.2, -6.4) -> (121.4, -6.4)
  line L8 (121.4, -6.4) -> (121.4, 0)
  line L9 (121.4, 0) -> (115, 0)
  line L10 (115, 0) -> (115, -3.2)
  line L11 (115, -3.2) -> (105, -3.2)
  line L12 (105, -3.2) -> (105, 0)
  line L13 (105, 0) -> (90.35, 0)
  line L14 (90.35, 0) -> (90.35, -3.2)
  line L15 (90.35, -3.2) -> (80.35, -3.2)
  line L16 (80.35, -3.2) -> (80.35, 0)
  line L17 (80.35, 0) -> (65.7, 0)
  line L18 (65.7, 0) -> (65.7, -3.2)
  line L19 (65.7, -3.2) -> (55.7, -3.2)
  line L20 (55.7, -3.2) -> (55.7, 0)
  line L21 (55.7, 0) -> (41.05, 0)
  line L22 (41.05, 0) -> (41.05, -3.2)
  line L23 (41.05, -3.2) -> (31.05, -3.2)
  line L24 (31.05, -3.2) -> (31.05, 0)
  line L25 (31.05, 0) -> (16.4, 0)
  line L26 (16.4, 0) -> (16.4, -3.2)
  line L27 (16.4, -3.2) -> (6.4, -3.2)
  line L28 (6.4, -3.2) -> (6.4, 0)
  line L29 (6.4, 0) -> (0, 0)
  line L30 (0, 0) -> (0, -6.4)
  line L31 (0, -6.4) -> (3.2, -6.4)
  line L32 (3.2, -6.4) -> (3.2, -16.4)
  line L33 (3.2, -16.4) -> (0, -16.4)
  line L34 (0, -16.4) -> (0, -22.3)
  line L35 (0, -22.3) -> (3.2, -22.3)
  line L36 (3.2, -22.3) -> (3.2, -32.3)
  line L37 (3.2, -32.3) -> (0, -32.3)
  line L38 (0, -32.3) -> (0, -38.2)
  line L39 (0, -38.2) -> (3.2, -38.2)
  line L40 (3.2, -38.2) -> (3.2, -48.2)
  line L41 (3.2, -48.2) -> (0, -48.2)
  line L42 (0, -48.2) -> (0, -54.1)
  line L43 (0, -54.1) -> (3.2, -54.1)
  line L44 (3.2, -54.1) -> (3.2, -64.1)
  line L45 (3.2, -64.1) -> (0, -64.1)
  line L46 (0, -64.1) -> (0, -70)
  line L47 (0, -70) -> (3.2, -70)
  line L48 (3.2, -70) -> (3.2, -80)
  line L49 (3.2, -80) -> (0, -80)
  line L50 (0, -80) -> (0, -86.4)
  line L51 (0, -86.4) -> (6.4, -86.4)
  line L52 (6.4, -86.4) -> (6.4, -83.2)
  line L53 (6.4, -83.2) -> (16.4, -83.2)
  line L54 (16.4, -83.2) -> (16.4, -86.4)
  line L55 (16.4, -86.4) -> (31.05, -86.4)
  line L56 (31.05, -86.4) -> (31.05, -83.2)
  line L57 (31.05, -83.2) -> (41.05, -83.2)
  line L58 (41.05, -83.2) -> (41.05, -86.4)
  line L59 (41.05, -86.4) -> (55.7, -86.4)
  line L60 (55.7, -86.4) -> (55.7, -83.2)
  line L61 (55.7, -83.2) -> (65.7, -83.2)
  line L62 (65.7, -83.2) -> (65.7, -86.4)
  line L63 (65.7, -86.4) -> (80.35, -86.4)
  line L64 (80.35, -86.4) -> (80.35, -83.2)
  line L65 (80.35, -83.2) -> (90.35, -83.2)
  line L66 (90.35, -83.2) -> (90.35, -86.4)
  line L67 (90.35, -86.4) -> (105, -86.4)
  line L68 (105, -86.4) -> (105, -83.2)
  line L69 (105, -83.2) -> (115, -83.2)
  line L70 (115, -83.2) -> (115, -86.4)
  line L71 (115, -86.4) -> (121.4, -86.4)
  line L72 (121.4, -86.4) -> (121.4, -80)
  line L73 (121.4, -80) -> (118.2, -80)
  line L74 (118.2, -80) -> (118.2, -70)
  line L75 (118.2, -70) -> (121.4, -70)
  line L76 (121.4, -70) -> (121.4, -64.1)
  line L77 (121.4, -64.1) -> (118.2, -64.1)
  line L78 (118.2, -64.1) -> (118.2, -54.1)
  line L79 (118.2, -54.1) -> (121.4, -54.1)
  line L80 (121.4, -54.1) -> (121.4, -48.2)
  line L81 (121.4, -48.2) -> (118.2, -48.2)
  line L82 (118.2, -48.2) -> (118.2, -38.2)
  line L83 (118.2, -38.2) -> (121.4, -38.2)
  line L84 (3.2, 0) -> (118.2, 0)
  line L85 (118.2, 0) -> (118.2, -3.2)
  line L86 (118.2, -3.2) -> (3.2, -3.2)
  line L87 (3.2, -3.2) -> (3.2, 0)
  dimension "d94" = 115
  dimension "d95" = 3.2
  constraint horizontal L84
  constraint vertical L85
  constraint horizontal L86
  constraint vertical L87
  constraint midpoint L29 L84.start
  measures "d94" distance of L84.start L84.end
  measures "d95" distance of L84.start L86.end
extrude "Extrude19" add sketch "Sketch18" along normal blind 2 contours L9 L10 L84 L85 L86 | L10 L11 L12 L84 L86 | L12 L13 L14 L84 L86 | L14 L15 L16 L84 L86 | L16 L17 L18 L84 L86 | L18 L19 L20 L84 L86 | L20 L21 L22 L84 L86 | L22 L23 L24 L84 L86 | L24 L25 L26 L84 L86 | L26 L27 L28 L84 L86 | L28 L29 L84 L86 L87 bodies 7
sketch "Sketch19" plane through (0, 0, 3.2) normal (0, 0, 1) x (-1, 0, 0)
  line L0 (-121.4, -32.3) -> (-121.4, -38.2)
  line L1 (-121.4, -38.2) -> (-118.2, -38.2)
  line L2 (-118.2, -38.2) -> (-118.2, -48.2)
  line L3 (-118.2, -48.2) -> (-121.4, -48.2)
  line L4 (-121.4, -48.2) -> (-121.4, -54.1)
  line L5 (-121.4, -54.1) -> (-118.2, -54.1)
  line L6 (-118.2, -54.1) -> (-118.2, -64.1)
  line L7 (-118.2, -64.1) -> (-121.4, -64.1)
  line L8 (-121.4, -64.1) -> (-121.4, -70)
  line L9 (-121.4, -70) -> (-118.2, -70)
  line L10 (-118.2, -70) -> (-118.2, -80)
  line L11 (-118.2, -80) -> (-121.4, -80)
  line L12 (-121.4, -80) -> (-121.4, -86.4)
  line L13 (-121.4, -86.4) -> (-115, -86.4)
  line L14 (-115, -86.4) -> (-115, -83.2)
  line L15 (-115, -83.2) -> (-105, -83.2)
  line L16 (-105, -83.2) -> (-105, -86.4)
  line L17 (-105, -86.4) -> (-90.35, -86.4)
  line L18 (-90.35, -86.4) -> (-90.35, -83.2)
  line L19 (-90.35, -83.2) -> (-80.35, -83.2)
  line L20 (-80.35, -83.2) -> (-80.35, -86.4)
  line L21 (-80.35, -86.4) -> (-65.7, -86.4)
  line L22 (-65.7, -86.4) -> (-65.7, -83.2)
  line L23 (-65.7, -83.2) -> (-55.7, -83.2)
  line L24 (-55.7, -83.2) -> (-55.7, -86.4)
  line L25 (-55.7, -86.4) -> (-41.05, -86.4)
  line L26 (-41.05, -86.4) -> (-41.05, -83.2)
  line L27 (-41.05, -83.2) -> (-31.05, -83.2)
  line L28 (-31.05, -83.2) -> (-31.05, -86.4)
  line L29 (-31.05, -86.4) -> (-16.4, -86.4)
  line L30 (-16.4, -86.4) -> (-16.4, -83.2)
  line L31 (-16.4, -83.2) -> (-6.4, -83.2)
  line L32 (-6.4, -83.2) -> (-6.4, -86.4)
  line L33 (-6.4, -86.4) -> (0, -86.4)
  line L34 (0, -86.4) -> (0, -80)
  line L35 (0, -80) -> (-3.2, -80)
  line L36 (-3.2, -80) -> (-3.2, -70)
  line L37 (-3.2, -70) -> (0, -70)
  line L38 (0, -70) -> (0, -64.1)
  line L39 (0, -64.1) -> (-3.2, -64.1)
  line L40 (-3.2, -64.1) -> (-3.2, -54.1)
  line L41 (-3.2, -54.1) -> (0, -54.1)
  line L42 (0, -54.1) -> (0, -48.2)
  line L43 (0, -48.2) -> (-3.2, -48.2)
  line L44 (-3.2, -48.2) -> (-3.2, -38.2)
  line L45 (-3.2, -38.2) -> (0, -38.2)
  line L46 (0, -38.2) -> (0, -32.3)
  line L47 (0, -32.3) -> (-3.2, -32.3)
  line L48 (-3.2, -32.3) -> (-3.2, -22.3)
  line L49 (-3.2, -22.3) -> (0, -22.3)
  line L50 (0, -22.3) -> (0, -16.4)
  line L51 (0, -16.4) -> (-3.2, -16.4)
  line L52 (-3.2, -16.4) -> (-3.2, -6.4)
  line L53 (-3.2, -6.4) -> (0, -6.4)
  line L54 (0, -6.4) -> (0, 0)
  line L55 (0, 0) -> (-6.4, 0)
  line L56 (-6.4, 0) -> (-6.4, -3.2)
  line L57 (-6.4, -3.2) -> (-16.4, -3.2)
  line L58 (-16.4, -3.2) -> (-16.4, 0)
  line L59 (-16.4, 0) -> (-31.05, 0)
  line L60 (-31.05, 0) -> (-31.05, -3.2)
  line L61 (-31.05, -3.2) -> (-41.05, -3.2)
  line L62 (-41.05, -3.2) -> (-41.05, 0)
  line L63 (-41.05, 0) -> (-55.7, 0)
  line L64 (-55.7, 0) -> (-55.7, -3.2)
  line L65 (-55.7, -3.2) -> (-65.7, -3.2)
  line L66 (-65.7, -3.2) -> (-65.7, 0)
  line L67 (-65.7, 0) -> (-80.35, 0)
  line L68 (-80.35, 0) -> (-80.35, -3.2)
  line L69 (-80.35, -3.2) -> (-90.35, -3.2)
  line L70 (-90.35, -3.2) -> (-90.35, 0)
  line L71 (-90.35, 0) -> (-105, 0)
  line L72 (-105, 0) -> (-105, -3.2)
  line L73 (-105, -3.2) -> (-115, -3.2)
  line L74 (-115, -3.2) -> (-115, 0)
  line L75 (-115, 0) -> (-121.4, 0)
  line L76 (-121.4, 0) -> (-121.4, -6.4)
  line L77 (-121.4, -6.4) -> (-118.2, -6.4)
  line L78 (-118.2, -6.4) -> (-118.2, -16.4)
  line L79 (-118.2, -16.4) -> (-121.4, -16.4)
  line L80 (-121.4, -16.4) -> (-121.4, -22.3)
  line L81 (-121.4, -22.3) -> (-118.2, -22.3)
  line L82 (-118.2, -22.3) -> (-118.2, -32.3)
  line L83 (-118.2, -32.3) -> (-121.4, -32.3)
  line L84 (-3.2, -86.4) -> (-118.2, -86.4)
  line L85 (-118.2, -86.4) -> (-118.2, -83.2)
  line L86 (-118.2, -83.2) -> (-3.2, -83.2)
  line L87 (-3.2, -83.2) -> (-3.2, -86.4)
  dimension "d98" = 115
  dimension "d99" = 3.2
  constraint horizontal L84
  constraint vertical L85
  constraint horizontal L86
  constraint vertical L87
  constraint midpoint L33 L84.start
  measures "d98" distance of L84.start L84.end
  measures "d99" distance of L84.start L86.end
extrude "Extrude20" add sketch "Sketch19" against normal blind 3.2 separate body contours L14 L15 L16 L84 L86 | L18 L19 L20 L84 L86 | L22 L23 L24 L84 L86 | L26 L27 L28 L84 L86 | L30 L31 L32 L84 L86 makes body 12 at (59.0333, 84.2667, 3.2) makes body 13 at (37.7167, 84.2667, 3.2) makes body 14 at (87.0167, 84.2667, 3.2) makes body 15 at (13.0667, 84.2667, 3.2) makes body 16 at (111.6667, 84.2667, 3.2)
extrude "Extrude21" add sketch "Sketch19" along normal blind 2 contours L13 L14 L84 L85 L86 | L14 L15 L16 L84 L86 | L16 L17 L18 L84 L86 | L18 L19 L20 L84 L86 | L20 L21 L22 L84 L86 | L22 L23 L24 L84 L86 | L24 L25 L26 L84 L86 | L26 L27 L28 L84 L86 | L28 L29 L30 L84 L86 | L30 L31 L32 L84 L86 | L32 L33 L84 L86 L87 bodies 12 13 14 15 16
sketch "Sketch20" plane through (0, 0, 0) normal (0, 0, -1) x (1, 0, 0)
  line L0 (121.4, -38.2) -> (121.4, -32.3)
  line L1 (121.4, -32.3) -> (118.2, -32.3)
  line L2 (118.2, -32.3) -> (118.2, -22.3)
  line L3 (118.2, -22.3) -> (121.4, -22.3)
  line L4 (121.4, -22.3) -> (121.4, -16.4)
  line L5 (121.4, -16.4) -> (118.2, -16.4)
  line L6 (118.2, -16.4) -> (118.2, -6.4)
  line L7 (118.2, -6.4) -> (121.4, -6.4)
  line L8 (121.4, -6.4) -> (121.4, 0)
  line L9 (121.4, 0) -> (115, 0)
  line L10 (115, 0) -> (115, -3.2)
  line L11 (115, -3.2) -> (105, -3.2)
  line L12 (105, -3.2) -> (105, 0)
  line L13 (105, 0) -> (90.35, 0)
  line L14 (90.35, 0) -> (90.35, -3.2)
  line L15 (90.35, -3.2) -> (80.35, -3.2)
  line L16 (80.35, -3.2) -> (80.35, 0)
  line L17 (80.35, 0) -> (65.7, 0)
  line L18 (65.7, 0) -> (65.7, -3.2)
  line L19 (65.7, -3.2) -> (55.7, -3.2)
  line L20 (55.7, -3.2) -> (55.7, 0)
  line L21 (55.7, 0) -> (41.05, 0)
  line L22 (41.05, 0) -> (41.05, -3.2)
  line L23 (41.05, -3.2) -> (31.05, -3.2)
  line L24 (31.05, -3.2) -> (31.05, 0)
  line L25 (31.05, 0) -> (16.4, 0)
  line L26 (16.4, 0) -> (16.4, -3.2)
  line L27 (16.4, -3.2) -> (6.4, -3.2)
  line L28 (6.4, -3.2) -> (6.4, 0)
  line L29 (6.4, 0) -> (0, 0)
  line L30 (0, 0) -> (0, -6.4)
  line L31 (0, -6.4) -> (3.2, -6.4)
  line L32 (3.2, -6.4) -> (3.2, -16.4)
  line L33 (3.2, -16.4) -> (0, -16.4)
  line L34 (0, -16.4) -> (0, -22.3)
  line L35 (0, -22.3) -> (3.2, -22.3)
  line L36 (3.2, -22.3) -> (3.2, -32.3)
  line L37 (3.2, -32.3) -> (0, -32.3)
  line L38 (0, -32.3) -> (0, -38.2)
  line L39 (0, -38.2) -> (3.2, -38.2)
  line L40 (3.2, -38.2) -> (3.2, -48.2)
  line L41 (3.2, -48.2) -> (0, -48.2)
  line L42 (0, -48.2) -> (0, -54.1)
  line L43 (0, -54.1) -> (3.2, -54.1)
  line L44 (3.2, -54.1) -> (3.2, -64.1)
  line L45 (3.2, -64.1) -> (0, -64.1)
  line L46 (0, -64.1) -> (0, -70)
  line L47 (0, -70) -> (3.2, -70)
  line L48 (3.2, -70) -> (3.2, -80)
  line L49 (3.2, -80) -> (0, -80)
  line L50 (0, -80) -> (0, -86.4)
  line L51 (0, -86.4) -> (6.4, -86.4)
  line L52 (6.4, -86.4) -> (6.4, -83.2)
  line L53 (6.4, -83.2) -> (16.4, -83.2)
  line L54 (16.4, -83.2) -> (16.4, -86.4)
  line L55 (16.4, -86.4) -> (31.05, -86.4)
  line L56 (31.05, -86.4) -> (31.05, -83.2)
  line L57 (31.05, -83.2) -> (41.05, -83.2)
  line L58 (41.05, -83.2) -> (41.05, -86.4)
  line L59 (41.05, -86.4) -> (55.7, -86.4)
  line L60 (55.7, -86.4) -> (55.7, -83.2)
  line L61 (55.7, -83.2) -> (65.7, -83.2)
  line L62 (65.7, -83.2) -> (65.7, -86.4)
  line L63 (65.7, -86.4) -> (80.35, -86.4)
  line L64 (80.35, -86.4) -> (80.35, -83.2)
  line L65 (80.35, -83.2) -> (90.35, -83.2)
  line L66 (90.35, -83.2) -> (90.35, -86.4)
  line L67 (90.35, -86.4) -> (105, -86.4)
  line L68 (105, -86.4) -> (105, -83.2)
  line L69 (105, -83.2) -> (115, -83.2)
  line L70 (115, -83.2) -> (115, -86.4)
  line L71 (115, -86.4) -> (121.4, -86.4)
  line L72 (121.4, -86.4) -> (121.4, -80)
  line L73 (121.4, -80) -> (118.2, -80)
  line L74 (118.2, -80) -> (118.2, -70)
  line L75 (118.2, -70) -> (121.4, -70)
  line L76 (121.4, -70) -> (121.4, -64.1)
  line L77 (121.4, -64.1) -> (118.2, -64.1)
  line L78 (118.2, -64.1) -> (118.2, -54.1)
  line L79 (118.2, -54.1) -> (121.4, -54.1)
  line L80 (121.4, -54.1) -> (121.4, -48.2)
  line L81 (121.4, -48.2) -> (118.2, -48.2)
  line L82 (118.2, -48.2) -> (118.2, -38.2)
  line L83 (118.2, -38.2) -> (121.4, -38.2)
  line L84 (3.2, -86.4) -> (118.2, -86.4)
  line L85 (118.2, -86.4) -> (118.2, -83.2)
  line L86 (118.2, -83.2) -> (3.2, -83.2)
  line L87 (3.2, -83.2) -> (3.2, -86.4)
  dimension "d104" = 115
  dimension "d105" = 3.2
  constraint horizontal L84
  constraint vertical L85
  constraint horizontal L86
  constraint vertical L87
  constraint midpoint L51 L84.start
  measures "d104" distance of L84.start L84.end
  measures "d105" distance of L84.start L86.end
extrude "Extrude22" add sketch "Sketch20" along normal blind 2 contours L70 L71 L84 L85 L86 | L68 L69 L70 L84 L86 | L66 L67 L68 L84 L86 | L64 L65 L66 L84 L86 | L62 L63 L64 L84 L86 | L60 L61 L62 L84 L86 | L58 L59 L60 L84 L86 | L56 L57 L58 L84 L86 | L54 L55 L56 L84 L86 | L52 L53 L54 L84 L86 | L51 L52 L84 L86 L87 bodies 12
sketch "Sketch21" plane through (0, 0, 3.2) normal (0, 0, 1) x (-1, 0, 0)
  line L0 (-121.4, -32.3) -> (-121.4, -38.2)
  line L1 (-121.4, -38.2) -> (-118.2, -38.2)
  line L2 (-118.2, -38.2) -> (-118.2, -48.2)
  line L3 (-118.2, -48.2) -> (-121.4, -48.2)
  line L4 (-121.4, -48.2) -> (-121.4, -54.1)
  line L5 (-121.4, -54.1) -> (-118.2, -54.1)
  line L6 (-118.2, -54.1) -> (-118.2, -64.1)
  line L7 (-118.2, -64.1) -> (-121.4, -64.1)
  line L8 (-121.4, -64.1) -> (-121.4, -70)
  line L9 (-121.4, -70) -> (-118.2, -70)
  line L10 (-118.2, -70) -> (-118.2, -80)
  line L11 (-118.2, -80) -> (-121.4, -80)
  line L12 (-121.4, -80) -> (-121.4, -86.4)
  line L13 (-121.4, -86.4) -> (-115, -86.4)
  line L14 (-115, -86.4) -> (-115, -83.2)
  line L15 (-115, -83.2) -> (-105, -83.2)
  line L16 (-105, -83.2) -> (-105, -86.4)
  line L17 (-105, -86.4) -> (-90.35, -86.4)
  line L18 (-90.35, -86.4) -> (-90.35, -83.2)
  line L19 (-90.35, -83.2) -> (-80.35, -83.2)
  line L20 (-80.35, -83.2) -> (-80.35, -86.4)
  line L21 (-80.35, -86.4) -> (-65.7, -86.4)
  line L22 (-65.7, -86.4) -> (-65.7, -83.2)
  line L23 (-65.7, -83.2) -> (-55.7, -83.2)
  line L24 (-55.7, -83.2) -> (-55.7, -86.4)
  line L25 (-55.7, -86.4) -> (-41.05, -86.4)
  line L26 (-41.05, -86.4) -> (-41.05, -83.2)
  line L27 (-41.05, -83.2) -> (-31.05, -83.2)
  line L28 (-31.05, -83.2) -> (-31.05, -86.4)
  line L29 (-31.05, -86.4) -> (-16.4, -86.4)
  line L30 (-16.4, -86.4) -> (-16.4, -83.2)
  line L31 (-16.4, -83.2) -> (-6.4, -83.2)
  line L32 (-6.4, -83.2) -> (-6.4, -86.4)
  line L33 (-6.4, -86.4) -> (0, -86.4)
  line L34 (0, -86.4) -> (0, -80)
  line L35 (0, -80) -> (-3.2, -80)
  line L36 (-3.2, -80) -> (-3.2, -70)
  line L37 (-3.2, -70) -> (0, -70)
  line L38 (0, -70) -> (0, -64.1)
  line L39 (0, -64.1) -> (-3.2, -64.1)
  line L40 (-3.2, -64.1) -> (-3.2, -54.1)
  line L41 (-3.2, -54.1) -> (0, -54.1)
  line L42 (0, -54.1) -> (0, -48.2)
  line L43 (0, -48.2) -> (-3.2, -48.2)
  line L44 (-3.2, -48.2) -> (-3.2, -38.2)
  line L45 (-3.2, -38.2) -> (0, -38.2)
  line L46 (0, -38.2) -> (0, -32.3)
  line L47 (0, -32.3) -> (-3.2, -32.3)
  line L48 (-3.2, -32.3) -> (-3.2, -22.3)
  line L49 (-3.2, -22.3) -> (0, -22.3)
  line L50 (0, -22.3) -> (0, -16.4)
  line L51 (0, -16.4) -> (-3.2, -16.4)
  line L52 (-3.2, -16.4) -> (-3.2, -6.4)
  line L53 (-3.2, -6.4) -> (0, -6.4)
  line L54 (0, -6.4) -> (0, 0)
  line L55 (0, 0) -> (-6.4, 0)
  line L56 (-6.4, 0) -> (-6.4, -3.2)
  line L57 (-6.4, -3.2) -> (-16.4, -3.2)
  line L58 (-16.4, -3.2) -> (-16.4, 0)
  line L59 (-16.4, 0) -> (-31.05, 0)
  line L60 (-31.05, 0) -> (-31.05, -3.2)
  line L61 (-31.05, -3.2) -> (-41.05, -3.2)
  line L62 (-41.05, -3.2) -> (-41.05, 0)
  line L63 (-41.05, 0) -> (-55.7, 0)
  line L64 (-55.7, 0) -> (-55.7, -3.2)
  line L65 (-55.7, -3.2) -> (-65.7, -3.2)
  line L66 (-65.7, -3.2) -> (-65.7, 0)
  line L67 (-65.7, 0) -> (-80.35, 0)
  line L68 (-80.35, 0) -> (-80.35, -3.2)
  line L69 (-80.35, -3.2) -> (-90.35, -3.2)
  line L70 (-90.35, -3.2) -> (-90.35, 0)
  line L71 (-90.35, 0) -> (-105, 0)
  line L72 (-105, 0) -> (-105, -3.2)
  line L73 (-105, -3.2) -> (-115, -3.2)
  line L74 (-115, -3.2) -> (-115, 0)
  line L75 (-115, 0) -> (-121.4, 0)
  line L76 (-121.4, 0) -> (-121.4, -6.4)
  line L77 (-121.4, -6.4) -> (-118.2, -6.4)
  line L78 (-118.2, -6.4) -> (-118.2, -16.4)
  line L79 (-118.2, -16.4) -> (-121.4, -16.4)
  line L80 (-121.4, -16.4) -> (-121.4, -22.3)
  line L81 (-121.4, -22.3) -> (-118.2, -22.3)
  line L82 (-118.2, -22.3) -> (-118.2, -32.3)
  line L83 (-118.2, -32.3) -> (-121.4, -32.3)
  line L84 (-121.4, 0) -> (-118.2, 0)
  line L85 (-118.2, 0) -> (-118.2, -86.4)
  line L86 (-118.2, -86.4) -> (-121.4, -86.4)
  line L87 (-121.4, -86.4) -> (-121.4, 0)
  dimension "d108" = 3.2
  dimension "d109" = 86.4
  constraint horizontal L84
  constraint vertical L85
  constraint horizontal L86
  constraint vertical L87
  constraint coincident L75.end L76.start
  measures "d108" distance of L75.end L84.end
  measures "d109" distance of L75.end L12.end
extrude "Extrude23" add sketch "Sketch21" against normal blind 3.2 separate body contours L81 L82 L83 L85 L87 | L1 L2 L3 L85 L87 | L77 L78 L79 L85 L87 | L5 L6 L7 L85 L87 | L9 L10 L11 L85 L87 makes body 17 at (120.3333, 44.8667, 3.2) makes body 18 at (120.3333, 25.6333, 3.2) makes body 19 at (120.3333, 57.4333, 3.2) makes body 20 at (120.3333, 9.7333, 3.2) makes body 21 at (118.2, 76.6667, 2.1333)
extrude "Extrude24" add sketch "Sketch21" along normal blind 2 contours L0 L1 L83 L85 L87 | L81 L82 L83 L85 L87 | L1 L2 L3 L85 L87 | L79 L80 L81 L85 L87 | L3 L4 L5 L85 L87 | L77 L78 L79 L85 L87 | L5 L6 L7 L85 L87 | L75 L76 L77 L84 L85 L87 | L7 L8 L9 L85 L87 | L9 L10 L11 L85 L87 | L11 L12 L13 L85 L86 L87 bodies 17 18 19 20 21
sketch "Sketch22" plane through (0, 0, 0) normal (0, 0, -1) x (1, 0, 0)
  line L0 (121.4, -38.2) -> (121.4, -32.3)
  line L1 (121.4, -32.3) -> (118.2, -32.3)
  line L2 (118.2, -32.3) -> (118.2, -22.3)
  line L3 (118.2, -22.3) -> (121.4, -22.3)
  line L4 (121.4, -22.3) -> (121.4, -16.4)
  line L5 (121.4, -16.4) -> (118.2, -16.4)
  line L6 (118.2, -16.4) -> (118.2, -6.4)
  line L7 (118.2, -6.4) -> (121.4, -6.4)
  line L8 (121.4, -6.4) -> (121.4, 0)
  line L9 (121.4, 0) -> (115, 0)
  line L10 (115, 0) -> (115, -3.2)
  line L11 (115, -3.2) -> (105, -3.2)
  line L12 (105, -3.2) -> (105, 0)
  line L13 (105, 0) -> (90.35, 0)
  line L14 (90.35, 0) -> (90.35, -3.2)
  line L15 (90.35, -3.2) -> (80.35, -3.2)
  line L16 (80.35, -3.2) -> (80.35, 0)
  line L17 (80.35, 0) -> (65.7, 0)
  line L18 (65.7, 0) -> (65.7, -3.2)
  line L19 (65.7, -3.2) -> (55.7, -3.2)
  line L20 (55.7, -3.2) -> (55.7, 0)
  line L21 (55.7, 0) -> (41.05, 0)
  line L22 (41.05, 0) -> (41.05, -3.2)
  line L23 (41.05, -3.2) -> (31.05, -3.2)
  line L24 (31.05, -3.2) -> (31.05, 0)
  line L25 (31.05, 0) -> (16.4, 0)
  line L26 (16.4, 0) -> (16.4, -3.2)
  line L27 (16.4, -3.2) -> (6.4, -3.2)
  line L28 (6.4, -3.2) -> (6.4, 0)
  line L29 (6.4, 0) -> (0, 0)
  line L30 (0, 0) -> (0, -6.4)
  line L31 (0, -6.4) -> (3.2, -6.4)
  line L32 (3.2, -6.4) -> (3.2, -16.4)
  line L33 (3.2, -16.4) -> (0, -16.4)
  line L34 (0, -16.4) -> (0, -22.3)
  line L35 (0, -22.3) -> (3.2, -22.3)
  line L36 (3.2, -22.3) -> (3.2, -32.3)
  line L37 (3.2, -32.3) -> (0, -32.3)
  line L38 (0, -32.3) -> (0, -38.2)
  line L39 (0, -38.2) -> (3.2, -38.2)
  line L40 (3.2, -38.2) -> (3.2, -48.2)
  line L41 (3.2, -48.2) -> (0, -48.2)
  line L42 (0, -48.2) -> (0, -54.1)
  line L43 (0, -54.1) -> (3.2, -54.1)
  line L44 (3.2, -54.1) -> (3.2, -64.1)
  line L45 (3.2, -64.1) -> (0, -64.1)
  line L46 (0, -64.1) -> (0, -70)
  line L47 (0, -70) -> (3.2, -70)
  line L48 (3.2, -70) -> (3.2, -80)
  line L49 (3.2, -80) -> (0, -80)
  line L50 (0, -80) -> (0, -86.4)
  line L51 (0, -86.4) -> (6.4, -86.4)
  line L52 (6.4, -86.4) -> (6.4, -83.2)
  line L53 (6.4, -83.2) -> (16.4, -83.2)
  line L54 (16.4, -83.2) -> (16.4, -86.4)
  line L55 (16.4, -86.4) -> (31.05, -86.4)
  line L56 (31.05, -86.4) -> (31.05, -83.2)
  line L57 (31.05, -83.2) -> (41.05, -83.2)
  line L58 (41.05, -83.2) -> (41.05, -86.4)
  line L59 (41.05, -86.4) -> (55.7, -86.4)
  line L60 (55.7, -86.4) -> (55.7, -83.2)
  line L61 (55.7, -83.2) -> (65.7, -83.2)
  line L62 (65.7, -83.2) -> (65.7, -86.4)
  line L63 (65.7, -86.4) -> (80.35, -86.4)
  line L64 (80.35, -86.4) -> (80.35, -83.2)
  line L65 (80.35, -83.2) -> (90.35, -83.2)
  line L66 (90.35, -83.2) -> (90.35, -86.4)
  line L67 (90.35, -86.4) -> (105, -86.4)
  line L68 (105, -86.4) -> (105, -83.2)
  line L69 (105, -83.2) -> (115, -83.2)
  line L70 (115, -83.2) -> (115, -86.4)
  line L71 (115, -86.4) -> (121.4, -86.4)
  line L72 (121.4, -86.4) -> (121.4, -80)
  line L73 (121.4, -80) -> (118.2, -80)
  line L74 (118.2, -80) -> (118.2, -70)
  line L75 (118.2, -70) -> (121.4, -70)
  line L76 (121.4, -70) -> (121.4, -64.1)
  line L77 (121.4, -64.1) -> (118.2, -64.1)
  line L78 (118.2, -64.1) -> (118.2, -54.1)
  line L79 (118.2, -54.1) -> (121.4, -54.1)
  line L80 (121.4, -54.1) -> (121.4, -48.2)
  line L81 (121.4, -48.2) -> (118.2, -48.2)
  line L82 (118.2, -48.2) -> (118.2, -38.2)
  line L83 (118.2, -38.2) -> (121.4, -38.2)
  line L84 (121.4, -86.4) -> (118.2, -86.4)
  line L85 (118.2, -86.4) -> (118.2, 0)
  line L86 (118.2, 0) -> (121.4, 0)
  line L87 (121.4, 0) -> (121.4, -86.4)
  dimension "d114" = 3.2
  dimension "d115" = 86.4
  constraint horizontal L84
  constraint vertical L85
  constraint horizontal L86
  constraint vertical L87
  constraint coincident L71.end L72.start
  measures "d114" distance of L71.end L84.end
  measures "d115" distance of L71.end L8.end
extrude "Extrude25" add sketch "Sketch22" along normal blind 2 contours L0 L1 L83 L85 L87 | L81 L82 L83 L85 L87 | L1 L2 L3 L85 L87 | L79 L80 L81 L85 L87 | L3 L4 L5 L85 L87 | L77 L78 L79 L85 L87 | L5 L6 L7 L85 L87 | L75 L76 L77 L85 L87 | L7 L8 L9 L85 L86 L87 | L73 L74 L75 L85 L87 | L71 L72 L73 L84 L85 L87 bodies 17